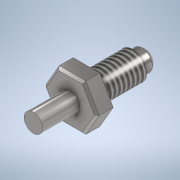
# Autodesk Inventor part: Thermocouple
Saved by Autodesk Inventor 2020 (Build 240168000, 168)
## iProperties
Created: 2020-06-17
Part Number: Thermocouple
Material: Steel
Document SubType Name: Modeling
Designer: Juan
Density: 7.85 g/cm^3
Appearance: Semi-Polished
Author: Juan
Autodesk Inventor part; units mm, degrees
ref_plane "YZ Plane" through (0, 0, 0) normal (1, 0, 0) x (0, 1, 0)
ref_plane "XZ Plane" through (0, 0, 0) normal (0, 1, 0) x (-1, 0, 0)
ref_plane "XY Plane" through (0, 0, 0) normal (0, 0, 1) x (1, 0, 0)
sketch "Sketch2" plane through (0, 0, 0) normal (1, 0, 0) x (0, 1, 0)
  line L0 (0, 0) -> (1, 0)
  line L1 (1, 0) -> (1, 1)
  line L2 (1, 1) -> (2.25, 1)
  line L3 (2.25, 1) -> (2.25, 3)
  line L4 (2.25, 3) -> (3, 3)
  line L5 (3, 3) -> (3, 13)
  line L6 (3, 13) -> (0, 13)
  line L7 (0, 13) -> (0, 0)
  arc A0 (1, 0) -> (2.25, 1) centre (0.8455, 1.4743) ccw
  dimension "d3" = 1
  dimension "d4" = 1
  dimension "d5" = 1.25
  dimension "d6" = 2
  dimension "d7" = 0.75
  dimension "d8" = 10
  dimension "d9" = 3
  constraints: 16 end point, 6 perpendicular, 2 point on circle, 1 centre point, 1 horizontal
  measures "d3" distance of L0.start L0.end
  measures "d4" distance of L0.end L1.end
  measures "d5" distance of L1.end L2.end
  measures "d6" distance of L2.end L3.end
  measures "d7" distance of L3.end L4.end
  measures "d8" distance of L4.end L5.end
  measures "d9" distance of L5.end L6.end
revolve "Revolution1" add sketch "Sketch2" angle 360 about axis through (0, 0, 13) along (0, 0, -1)
thread "Thread1" size "M6x1" class "6g" standard "ANSI Metric M Profile" full length
sketch "Sketch3" plane through (0, 0, 13) normal (0, 0, 1) x (1, 0, 0)
  line L0 (2.8868, 5) -> (5.7735, 0)
  line L1 (5.7735, 0) -> (2.8868, -5)
  line L2 (2.8868, -5) -> (-2.8868, -5)
  line L3 (-2.8868, -5) -> (-5.7735, 0)
  line L4 (-5.7735, 0) -> (-2.8868, 5)
  line L5 (-2.8868, 5) -> (2.8868, 5)
  point P0 (0, 0)
  point P1 (0, 0)
  dimension "d13" = 10
  constraints: 12 end point, 1 coincident, 13 other
  measures "d13" distance between parallel lines of L2 L5
extrude "Extrusion2" add sketch "Sketch3" along normal blind 3.5
chamfer "Chamfer1" distance 0.5 angle 45 6 edges at (0, 5, 16.5) (4.3301, 2.5, 16.5) (4.3301, -2.5, 16.5) (0, -5, 16.5) (-4.3301, -2.5, 16.5) (-4.3301, 2.5, 16.5)
sketch "Sketch4" plane through (0, 0, 16.5) normal (0, 0, 1) x (1, 0, 0)
  circle A0 centre (0, 0) radius 2
  dimension "d19" = 4
  constraints: 1 centre point, 1 coincident
  measures "d19" diameter of A0
extrude "Extrusion3" add sketch "Sketch4" along normal blind 8
body "Solid2"
